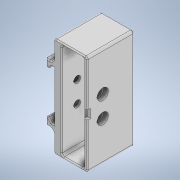
# Autodesk Inventor part: EndSwitchHousing_v02
Saved by Autodesk Inventor 2020 (Build 240168000, 168)
## iProperties
Created: 2020-02-12
Part Number: EndSwitchHousing_v02
Material: Generic
Document SubType Name: Modeling
Designer: Timo
Density: 1 g/cm^3
Appearance: Default
Author: Timo
Autodesk Inventor part; units mm, degrees
ref_plane "YZ Plane" through (0, 0, 0) normal (1, 0, 0) x (0, 1, 0)
ref_plane "XZ Plane" through (0, 0, 0) normal (0, 1, 0) x (-1, 0, 0)
ref_plane "XY Plane" through (0, 0, 0) normal (0, 0, 1) x (1, 0, 0)
sketch "Sketch1" plane through (0, 0, 0) normal (1, 0, 0) x (0, 1, 0)
  line L0 (-22.5, 0) -> (22.5, 0)
  line L1 (22.5, 0) -> (22.5, 21)
  line L2 (22.5, 21) -> (-22.5, 21)
  line L3 (-22.5, 21) -> (-22.5, 0)
  point P0 (0, 0)
  point P1 (0, 0)
  dimension "d0" = 45
  dimension "d1" = 21
  constraints: 8 end point, 2 parallel, 1 coincident, 1 horizontal, 1 midpoint, 1 perpendicular
  measures "d0" distance of L1.end L2.end
  measures "d1" distance of L0.end L1.end
extrude "Extrusion1" add sketch "Sketch1" along normal blind 1
sketch "Sketch2" plane through (1, 0, 0) normal (1, 0, 0) x (0, 0, -1)
  line L0 (0, -22.5) -> (0, 22.5) projected
  line L1 (-21, -22.5) -> (0, -22.5) projected
  line L2 (0, 22.5) -> (-2, 22.5)
  line L3 (-2, 22.5) -> (-2, -22.5)
  line L4 (-2, -22.5) -> (0, -22.5)
  line L5 (0, -22.5) -> (0, 22.5)
  line L6 (-21, 22.5) -> (-21, -22.5) projected
  line L7 (-21, 22.5) -> (-2, 22.5)
  line L8 (-2, 22.5) -> (-2, 21.5)
  line L9 (-2, 21.5) -> (-21, 21.5)
  line L10 (-21, 21.5) -> (-21, 22.5)
  line L11 (-2, -22.5) -> (-21, -22.5)
  line L12 (-21, -22.5) -> (-21, -21.5)
  line L13 (-21, -21.5) -> (-2, -21.5)
  line L14 (-2, -21.5) -> (-2, -22.5)
  point P0 (0, 0)
  point P1 (-2, -21.5)
  point P2 (-21, -21.5)
  dimension "d4" = 2
  dimension "d12" = 1
  dimension "d13" = 1
  constraints: 24 end point, 6 parallel, 3 horizontal, 3 perpendicular, 3 point on line
  measures "d4" distance of L0.end L2.end
  measures "d12" distance between parallel lines of L7 L9
  measures "d13" distance between parallel lines of L1 L13
extrude "Extrusion2" add sketch "Sketch2" along normal blind 10 contours L1 L3 L2 L0 | L1 L6 L13 L3 | L3 L9 L6 L7
sketch "Sketch6" plane through (0, 0, 0) normal (-1, 0, 0) x (0, 0, 1)
  line L0 (0, -22.5) -> (0, 22.5) projected
  line L1 (21, 22.5) -> (21, -22.5) projected
  line L2 (0, 22.5) -> (21, 22.5)
  line L3 (21, 22.5) -> (21, -22.5)
  line L4 (21, -22.5) -> (0, -22.5)
  line L5 (0, -22.5) -> (0, 22.5)
  point P0 (0, 0)
  point P1 (0, -22.5)
  point P2 (21, 22.5)
  constraints: 8 end point, 2 parallel, 1 horizontal, 1 perpendicular
extrude "Extrusion5" add sketch "Sketch6" along normal blind 2.5
sketch "Sketch3" plane through (1, 0, 0) normal (1, 0, 0) x (0, 0, -1)
  circle A0 centre (-9, 15.5) radius 1.5
  line L0 (-2, 21.5) -> (-2, -21.5) projected
  line L1 (-10.25, 16.3292) -> (-10.8, 15.5)
  line L2 (-10.8, 15.5) -> (-10.25, 14.6708)
  line L3 (-10.8, 15.5) -> (-9, 15.5) construction
  line L4 (-20.1514, 10.75) -> (4.4488, 10.75) construction
  line L5 (-21, 21.5) -> (-2, 21.5) construction
  circle A1 centre (-9, 6) radius 1.5
  line L6 (-10.25, 5.1708) -> (-10.8, 6)
  line L7 (-10.8, 6) -> (-10.25, 6.8292)
  point P0 (0, 0)
  point P1 (-1, 15)
  point P2 (-1, -15)
  point P3 (-2, -21.5)
  dimension "d8" = 3
  dimension "d9" = 7
  dimension "d14" = 1.8
  dimension "d29" = 6
  dimension "d30" = 4.75
  dimension "d31" = 10.75
  constraints: 12 end point, 4 point on circle, 3 tangent, 2 centre point, 2 horizontal, 4 other
  measures "d8" diameter of A0
  measures "d14" distance of L3.end L1.end
  measures "d29" distance from line of L5 L3.end
  measures "d30" distance from line of L3.end L4
  measures "d31" distance between parallel lines of L5 L4
extrude "Extrusion3" [suppressed]
sketch "Sketch7" plane through (-2.5, 0, 0) normal (-1, 0, 0) x (0, 0, 1)
  arc A0 (9.25, 16.3292) -> (9.25, 14.6708) centre (8, 15.5) ccw projected
  line L0 (10.9445, 15.5) -> (9.4722, 12.95)
  line L1 (9.4722, 12.95) -> (6.5278, 12.95)
  line L2 (6.5278, 12.95) -> (5.0555, 15.5)
  line L3 (5.0555, 15.5) -> (6.5278, 18.05)
  line L4 (6.5278, 18.05) -> (9.4722, 18.05)
  line L5 (9.4722, 18.05) -> (10.9445, 15.5)
  arc A1 (9.25, 6.8292) -> (9.25, 5.1708) centre (8, 6) ccw projected
  line L6 (10.9445, 6) -> (9.4722, 3.45)
  line L7 (9.4722, 3.45) -> (6.5278, 3.45)
  line L8 (6.5278, 3.45) -> (5.0555, 6)
  line L9 (5.0555, 6) -> (6.5278, 8.55)
  line L10 (6.5278, 8.55) -> (9.4722, 8.55)
  line L11 (9.4722, 8.55) -> (10.9445, 6)
  point P0 (0, 0)
  point P1 (8, 12.95)
  dimension "d36" = 5.1
  dimension "d37" = 5.1
  constraints: 24 end point, 2 coincident, 2 horizontal, 1 midpoint, 26 other
  measures "d36" distance between parallel lines of L10 L7
  measures "d37" distance between parallel lines of L4 L1
extrude "Extrusion6" [suppressed]
sketch "Sketch13" plane through (11, 0, 0) normal (1, 0, 0) x (0, 0, -1)
  line L0 (-21, -22.5) -> (0, -22.5) projected
  line L1 (-21, -22.5) -> (0, -22.5)
  line L2 (0, -22.5) -> (0, 22.5)
  line L3 (0, 22.5) -> (-21, 22.5)
  line L4 (-21, 22.5) -> (-21, -22.5)
  point P0 (0, 0)
  point P1 (0, -22.5)
  constraints: 8 end point, 2 parallel, 1 horizontal, 1 perpendicular
extrude "Extrusion9" add sketch "Sketch13" along normal blind 1.5
sketch "Sketch14" plane through (1, -21.5, 2) normal (0, 0, 1) x (1, 0, 0)
  circle A0 centre (5, 38) radius 3.15
  circle A1 centre (5, 5) radius 3.15
  line L0 (-3.2, 21.5) -> (12.2, 21.5) projected
  line L1 (5, 38) -> (5, 5) construction
  line L2 (0, 43) -> (0, 0) construction
  line L3 (10, 43) -> (10, 0) construction
  circle A2 centre (5, 38) radius 5 construction
  line L4 (0, 43) -> (10, 43) construction
  point P0 (-1, 21.5)
  dimension "d64" = 6.3
  dimension "d65" = 33
  dimension "d66" = 16.5
  dimension "d67" = 5
  dimension "d68" = 5
  dimension "d69" = 10
  constraints: 3 centre point, 2 end point, 1 coincident, 1 equal radius, 1 tangent, 1 vertical
  measures "d64" diameter of A0
  measures "d65" distance of L1.end L1.start
  measures "d66" distance from line of L1.start L0
  measures "d67" distance between parallel lines of L2 L1
  measures "d68" distance between parallel lines of L3 L1
  measures "d69" diameter of A2
extrude "Extrusion10" cut sketch "Sketch14" against normal through all
sketch "Sketch17" plane through (1, -21.5, 2) normal (0, 0, 1) x (1, 0, 0)
  line L0 (10, 43) -> (10, 0) projected
  line L1 (10, 11.6) -> (6.5, 11.6)
  line L2 (6.5, 11.6) -> (6.5, 31.4)
  line L3 (6.5, 31.4) -> (10, 31.4)
  line L4 (10, 31.4) -> (10, 11.6)
  line L5 (0, 43) -> (0, 0) projected
  line L6 (-3.2, 21.5) -> (12.2, 21.5) projected
  point P0 (-1, 21.5)
  point P1 (6.5, 21.5)
  dimension "d80" = 19.8
  dimension "d81" = 6.5
  constraints: 8 end point, 2 parallel, 2 point on line, 1 horizontal, 1 midpoint, 1 perpendicular
  measures "d80" distance of L1.end L2.end
  measures "d81" distance between parallel lines of L5 L2
extrude "Extrusion12" add sketch "Sketch17" along normal blind 15
sketch "Sketch15" plane through (12.5, 0, 0) normal (1, 0, 0) x (0, 0, -1)
  line L0 (-21, 21.5) -> (-21, -21.5) construction
  line L1 (-21, 9.9) -> (-11.2, 9.9) construction
  line L2 (-11.2, 9.9) -> (-11.2, -9.9) construction
  line L3 (-11.2, -9.9) -> (-21, -9.9) construction
  line L4 (-21, -9.9) -> (-21, 9.9) construction
  line L5 (4.2, 0) -> (-25.2, 0) construction
  circle A0 centre (-14, 4.75) radius 1.5
  circle A1 centre (-14, -4.75) radius 1.5
  line L6 (-14, 4.75) -> (-14, -4.75) construction
  line L7 (-15.2857, 5.5226) -> (-15.75, 4.75)
  line L8 (-15.75, 4.75) -> (-15.2857, 3.9774)
  line L9 (-15.2857, -3.9774) -> (-15.75, -4.75)
  line L10 (-15.75, -4.75) -> (-15.2857, -5.5226)
  line L11 (-15.75, 4.75) -> (-14, 4.75) construction
  point P0 (0, 0)
  point P1 (-11.2, 0)
  dimension "d72" = 9.8
  dimension "d73" = 19.8
  dimension "d74" = 2.8
  dimension "d75" = 3
  dimension "d76" = 9.5
  dimension "d77" = 1.75
  constraints: 20 end point, 4 point on circle, 4 tangent, 3 parallel, 2 centre point, 2 horizontal, 2 point on line, 1 equal radius, 1 midpoint, 1 perpendicular, 1 vertical, 3 other
  measures "d72" distance of L1.start L1.end
  measures "d73" distance of L1.end L2.end
  measures "d74" distance between parallel lines of L6 L2
  measures "d75" diameter of A0
  measures "d76" distance of L6.end L6.start
  measures "d77" distance of L6.start L7.end
extrude "Extrusion11" cut sketch "Sketch15" against normal through all
sketch "Sketch18" plane through (-2.5, 0, 0) normal (-1, 0, 0) x (0, 0, 1)
  arc A0 (15.2857, 5.5226) -> (15.2857, 3.9774) centre (14, 4.75) ccw projected
  line L0 (16.9445, 4.75) -> (15.4722, 2.2)
  line L1 (15.4722, 2.2) -> (12.5278, 2.2)
  line L2 (12.5278, 2.2) -> (11.0555, 4.75)
  line L3 (11.0555, 4.75) -> (12.5278, 7.3)
  line L4 (12.5278, 7.3) -> (15.4722, 7.3)
  line L5 (15.4722, 7.3) -> (16.9445, 4.75)
  arc A1 (15.2857, -3.9774) -> (15.2857, -5.5226) centre (14, -4.75) ccw projected
  line L6 (16.9445, -4.75) -> (15.4722, -7.3)
  line L7 (15.4722, -7.3) -> (12.5278, -7.3)
  line L8 (12.5278, -7.3) -> (11.0555, -4.75)
  line L9 (11.0555, -4.75) -> (12.5278, -2.2)
  line L10 (12.5278, -2.2) -> (15.4722, -2.2)
  line L11 (15.4722, -2.2) -> (16.9445, -4.75)
  point P0 (0, 0)
  dimension "d85" = 5.1
  constraints: 24 end point, 2 coincident, 2 horizontal, 1 parallel, 26 other
  measures "d85" distance between parallel lines of L4 L1
extrude "Extrusion13" cut sketch "Sketch18" against normal blind 2.5
sketch "Sketch19" plane through (12.5, 0, 0) normal (1, 0, 0) x (0, 0, -1)
  arc A0 (-15.2857, -5.5226) -> (-15.2857, -3.9774) centre (-14, -4.75) ccw projected
  circle A1 centre (-14, -4.75) radius 2.5
  arc A2 (-15.2857, 3.9774) -> (-15.2857, 5.5226) centre (-14, 4.75) ccw projected
  circle A3 centre (-14, 4.75) radius 2.5
  line L0 (-16.2727, -5.7915) -> (-16.75, -4.75)
  line L1 (-16.75, -4.75) -> (-16.2727, -3.7085)
  line L2 (-16.2727, 3.7085) -> (-16.75, 4.75)
  line L3 (-16.75, 4.75) -> (-16.2727, 5.7915)
  line L4 (-16.75, -4.75) -> (-14, -4.75) construction
  line L5 (4.2, 0) -> (-25.2, 0) construction
  point P0 (0, 0)
  dimension "d90" = 5
  dimension "d91" = 2.75
  constraints: 10 end point, 4 point on circle, 2 centre point, 2 coincident, 2 tangent, 1 equal radius, 1 horizontal, 2 other
  measures "d90" diameter of A1
  measures "d91" distance of A1.centre L0.end
extrude "Extrusion14" cut sketch "Sketch19" against normal blind 2
sketch "Sketch10" plane through (-2.5, -22.5, 21) normal (0, 0, 1) x (1, 0, 0)
  line L0 (0, 35.5) -> (-3.5, 35.5)
  line L1 (-3.5, 35.5) -> (-3.5, 32)
  line L2 (-3.5, 32) -> (-2.5, 32)
  line L3 (-2.5, 32) -> (-1, 33.5)
  line L4 (-1, 33.5) -> (0, 33.5)
  line L5 (0, 35.5) -> (0, 33.5)
  line L6 (-6.9, 22.5) -> (16.9, 22.5) projected
  line L7 (0, 0) -> (0, 45) projected
  point P0 (2.5, 22.5)
  dimension "d42" = 3.5
  dimension "d43" = 1
  dimension "d44" = 1
  dimension "d45" = 3.5
  dimension "d46" = 135
  dimension "d47" = 2
  dimension "d84" = 13
  constraints: 12 end point, 2 horizontal, 2 perpendicular, 1 point on line
  measures "d42" distance of L0.start L0.end
  measures "d43" distance of L3.end L4.end
  measures "d44" distance of L1.end L2.end
  measures "d45" distance of L0.end L1.end
  measures "d46" angle of L2 L3
  measures "d47" distance between parallel lines of L0 L4
  measures "d84" distance between parallel lines of L0 L6
extrude "Extrusion7" add sketch "Sketch10" against normal up to surface (21 mm away)
mirror "Mirror2" about plane through (0, 0, 0) normal (0, 1, 0) of "Extrusion7"
fillet "Fillet2" radius 1 12 edges at (12.5, -22.5, 10.5) (12.5, 22.5, 10.5) (-2.5, 22.5, 10.5) (-2.5, -22.5, 10.5) (1, -21.5, 11.5) (11, -21.5, 11.5) (11, 9.9, 9.5) (7.5, 9.9, 9.5) (7.5, -9.9, 9.5) (11, -9.9, 9.5) (1, 21.5, 11.5) (11, 21.5, 11.5)
fillet "Fillet3" radius 2 2 edges at (-2.5, 13, 10.5) (-2.5, -13, 10.5)
chamfer "Chamfer1" distance 0.5 angle 45 52 edges at (6, 21.5, 21) (10.7071, 21.2071, 21) (11, 0, 21) (10.7071, -21.2071, 21) (6, -21.5, 21) (1.2929, -21.2071, 21) (1, 0, 21) (1.2929, 21.2071, 21) (5, 22.5, 0) (-2.2071, 22.2071, 0) (-2.5, 18.25, 0) (-3.0858, 13.5858, 0) (-5.25, 13, 0) (12.2071, 22.2071, 0) (12.5, 0, 0) (12.2071, -22.2071, 0) (5, -22.5, 0) (-2.2071, -22.2071, 0) (-2.5, -18.25, 0) (-3.0858, -13.5858, 0) (-5.25, -13, 0) (-2.5, 0, 0) (-2.5, 0, 21) (-5.25, 13, 21) (-3.0858, 13.5858, 21) (-2.5, 18.25, 21) (-2.2071, 22.2071, 21) (5, 22.5, 21) (12.2071, 22.2071, 21) (12.5, 0, 21) (12.2071, -22.2071, 21) (5, -22.5, 21) (-2.2071, -22.2071, 21) (-2.5, -18.25, 21) (-3.0858, -13.5858, 21) (-5.25, -13, 21) (-3, -11, 0) (-4.25, -10.25, 0) (-5.5, -9.5, 0) (-6, -11.25, 0) (-3, 11, 0) (-4.25, 10.25, 0) (-5.5, 9.5, 0) (-6, 11.25, 0) (-3, -11, 21) (-4.25, -10.25, 21) (-5.5, -9.5, 21) (-6, -11.25, 21) (-6, 11.25, 21) (-5.5, 9.5, 21) (-4.25, 10.25, 21) (-3, 11, 21)
fillet "Fillet1" radius 0.5 2 edges at (-6, 9.5, 10.5) (-6, -9.5, 10.5)
sketch "Sketch20" plane through (12.5, 0, 0) normal (1, 0, 0) x (0, 0, -1)
  line L0 (-21, -2) -> (-19.5, -2)
  line L1 (-19.5, -2) -> (-19.5, 2)
  line L2 (-19.5, 2) -> (-21, 2)
  line L3 (-21, 2) -> (-21, -2)
  line L4 (-21, 21.5) -> (-21, -21.5) projected
  point P0 (0, 0)
  point P1 (-21, 0)
  dimension "d94" = 4
  dimension "d95" = 1.5
  constraints: 8 end point, 2 midpoint, 2 parallel, 1 horizontal, 1 perpendicular
  measures "d94" distance of L2.end L0.start
  measures "d95" distance of L1.end L2.end
extrude "Extrusion15" cut sketch "Sketch20" against normal up to next
equation "\"d13\" = d12"
equation "\"d30\" = 0.5 * d7"
equation "\"d37\" = d36"
equation "\"d66\" = 0.5 * d65"
equation "\"d67\" = d68"
equation "\"d7\" = 9.5"
body "Solid1"
